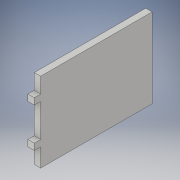
# Autodesk Inventor part: sidestandforservoclamp
Saved by Autodesk Inventor 2019 (Build 230136000, 136)
## iProperties
Created: 2020-02-29
Part Number: sidestandforservoclamp
Material: Generic
Document SubType Name: Modeling
Designer: Hp
Density: 1 g/cm^3
Appearance: Default
Author: Hp
Autodesk Inventor part; units mm, degrees
ref_plane "YZ Plane" through (0, 0, 0) normal (1, 0, 0) x (0, 1, 0)
ref_plane "XZ Plane" through (0, 0, 0) normal (0, 1, 0) x (-1, 0, 0)
ref_plane "XY Plane" through (0, 0, 0) normal (0, 0, 1) x (1, 0, 0)
sketch "Sketch1" plane through (0, 0, 0) normal (1, 0, 0) x (0, 1, 0)
  line L0 (10.6126, 22.7394) -> (-14.3874, 22.7394)
  line L1 (-14.3874, 22.7394) -> (-14.3874, -12.2606)
  line L2 (-14.3874, -12.2606) -> (10.6126, -12.2606)
  line L3 (10.6126, -12.2606) -> (10.6126, 22.7394)
  line L4 (5.7696, 24.7394) -> (3.7696, 24.7394)
  line L5 (3.7696, 24.7394) -> (3.7696, 22.7394)
  line L6 (3.7696, 22.7394) -> (5.7696, 22.7394)
  line L7 (5.7696, 22.7394) -> (5.7696, 24.7394)
  line L8 (-6.5839, 24.7394) -> (-8.5839, 24.7394)
  line L9 (-8.5839, 24.7394) -> (-8.5839, 22.7394)
  line L10 (-8.5839, 22.7394) -> (-6.5839, 22.7394)
  line L11 (-6.5839, 22.7394) -> (-6.5839, 24.7394)
  line L12 (3.7696, 22.7394) -> (-6.5839, 22.7394)
  point P0 (0, 0)
  dimension "d0" = 25
  dimension "d1" = 35
  dimension "d2" = 2
  dimension "d3" = 2
  dimension "d4" = 2
  dimension "d5" = 2
  constraints: 26 end point, 6 parallel, 3 horizontal, 3 perpendicular, 1 collinear, 1 point on line
  measures "d0" distance of L2.end L1.end
  measures "d1" distance of L1.end L0.end
  measures "d2" distance of L6.end L5.end
  measures "d3" distance of L5.end L4.end
  measures "d4" distance of L10.end L9.end
  measures "d5" distance of L9.end L8.end
extrude "Extrusion1" add sketch "Sketch1" along normal blind 2
body "Solid1"
